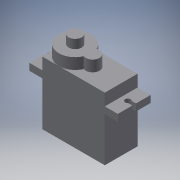
# Autodesk Inventor part: sg90
Saved by Autodesk Inventor 2018 (Build 220112000, 112)
## iProperties
Created: 2017-12-22
Part Number: sg90
Material: Generic
Document SubType Name: Modeling
Designer: Nirant Ramakuru
Density: 1 g/cm^3
Appearance: Default
Author: Nirant Ramakuru
Autodesk Inventor part; units mm, degrees
ref_plane "YZ Plane" through (0, 0, 0) normal (1, 0, 0) x (0, 1, 0)
ref_plane "XZ Plane" through (0, 0, 0) normal (0, 1, 0) x (-1, 0, 0)
ref_plane "XY Plane" through (0, 0, 0) normal (0, 0, 1) x (1, 0, 0)
sketch "Sketch1" plane through (0, 0, 0) normal (0, 1, 0) x (-1, 0, 0)
  line L0 (0, 0) -> (22.5, 0)
  line L1 (22.5, 0) -> (22.5, -11.8)
  line L2 (22.5, -11.8) -> (0, -11.8)
  line L3 (0, -11.8) -> (0, 0)
  dimension "d0" = 22.5
  dimension "d1" = 11.8
  constraints: 8 end point, 2 parallel, 1 horizontal, 1 perpendicular
  measures "d0" distance of L1.end L2.end
  measures "d1" distance of L0.end L1.end
extrude "Extrusion1" add sketch "Sketch1" along normal blind 22.7
sketch "Sketch2" plane through (0, 22.7, 0) normal (0, 1, 0) x (1, 0, 0)
  point P0 (0, 0)
sketch "Sketch3" plane through (0, 22.7, 0) normal (0, 1, 0) x (1, 0, 0)
  line L0 (-22.5, 0) -> (0, 0) projected
  line L1 (-18.5174, 0) -> (-18.5174, 5.9)
  line L2 (-18.5174, 0) -> (-12.6174, 0) construction
  line L3 (-22.5, 11.8) -> (-22.5, 0) projected
  line L4 (-22.5, 5.9) -> (-16.6, 5.9)
  circle A0 centre (-16.6, 5.9) radius 5.9
  dimension "d4" = 5.9
  dimension "d5" = 90
  dimension "d6" = 5.9
  constraints: 6 end point, 3 perpendicular, 1 coincident, 1 horizontal, 1 horizontal alignment, 1 midpoint, 1 point on line, 2 other
  measures "d4" distance of L1.start L1.end
  measures "d5" angle of L2 L1
  measures "d6" distance of L4.start L4.end
extrude "Extrusion2" add sketch "Sketch3" along normal blind 4 contours A0 L1 L4 | L4 L1 A0
sketch "Sketch4" plane through (0, 0, 0) normal (1, 0, 0) x (0, 0, -1)
  line L0 (0, 0) -> (11.8, 0) projected
  line L1 (5.9, 0) -> (5.9, 15.9)
  line L2 (0, 0) -> (0, 22.7) projected
  line L3 (11.8, 0) -> (11.8, 22.7) projected
  line L4 (0, 15.9) -> (11.8, 15.9)
  line L5 (11.8, 15.9) -> (11.8, 18.4)
  line L6 (11.8, 18.4) -> (0, 18.4)
  line L7 (0, 18.4) -> (0, 15.9)
  dimension "d9" = 15.9
  dimension "d10" = 2.5
  constraints: 10 end point, 2 parallel, 2 point on line, 1 horizontal, 1 midpoint, 1 perpendicular, 1 vertical
  measures "d9" distance of L1.start L1.end
  measures "d10" distance of L5.end L4.end
sketch "Sketch5" plane through (-22.5, 0, -11.8) normal (-1, 0, 0) x (0, 0, 1)
  line L0 (11.8, 0) -> (0, 0) projected
  line L1 (5.9, 0) -> (5.9, 15.9)
  line L2 (0, 0) -> (0, 22.7) projected
  line L3 (11.8, 0) -> (11.8, 22.7) projected
  line L4 (0, 15.9) -> (11.8, 15.9)
  line L5 (11.8, 15.9) -> (11.8, 18.4)
  line L6 (11.8, 18.4) -> (0, 18.4)
  line L7 (0, 18.4) -> (0, 15.9)
  dimension "d11" = 15.9
  dimension "d12" = 2.5
  constraints: 10 end point, 2 parallel, 2 point on line, 1 horizontal, 1 midpoint, 1 perpendicular, 1 vertical
  measures "d11" distance of L1.start L1.end
  measures "d12" distance of L5.end L4.end
extrude "Extrusion3" add sketch "Sketch5" along normal blind 4.7 contours L4 L2 L6 L3
extrude "Extrusion4" add sketch "Sketch4" along normal blind 4.7 contours L2 L6 L3 L4
sketch "Sketch6" plane through (-16.6, 26.7, -5.9) normal (0, 1, 0) x (1, 0, 0)
  point P0 (16.6, -5.9)
sketch "Sketch7" plane through (-16.6, 26.7, -5.9) normal (0, 1, 0) x (1, 0, 0)
  circle A0 centre (0, 0) radius 2.35
  point P0 (16.6, -5.9)
  dimension "d17" = 4.7
  constraints: 1 centre point, 1 coincident
  measures "d17" diameter of A0
extrude "Extrusion5" add sketch "Sketch7" along normal blind 3.2
sketch "Sketch8" plane through (0, 22.7, 0) normal (0, 1, 0) x (1, 0, 0)
  point P0 (0, 0)
sketch "Sketch9" plane through (-16.6, 26.7, -5.9) normal (0, 1, 0) x (1, 0, 0)
  line L0 (0, 0) -> (6.3, 0)
  point P0 (16.6, -5.9)
  dimension "d20" = 6.3
  constraints: 2 end point, 1 horizontal
  measures "d20" distance of L0.start L0.end
sketch "Sketch10" plane through (-16.6, 26.7, -5.9) normal (0, 1, 0) x (1, 0, 0)
  circle A0 centre (6.3, 0) radius 2.5
  point P0 (16.6, -5.9)
  dimension "d21" = 5
  constraints: 1 centre point
  measures "d21" diameter of A0
extrude "Extrusion6" add sketch "Sketch10" against normal blind 4
sketch "Sketch11" plane through (0, 18.4, 0) normal (0, 1, 0) x (1, 0, 0)
  line L0 (4.7, 0) -> (4.7, 11.8) projected
  line L1 (4.7, 5.9) -> (2.4, 5.9)
  circle A0 centre (2.4, 5.9) radius 1
  line L2 (0.1, 5.25) -> (4.7, 5.25)
  line L3 (4.7, 5.25) -> (4.7, 6.55)
  line L4 (4.7, 6.55) -> (0.1, 6.55)
  line L5 (0.1, 6.55) -> (0.1, 5.25)
  line L6 (2.4, 5.25) -> (2.4, 6.55)
  point P0 (0, 0)
  dimension "d24" = 2.3
  dimension "d25" = 2
  dimension "d26" = 1.3
  constraints: 12 end point, 3 midpoint, 2 horizontal, 2 parallel, 1 centre point, 1 coincident, 1 perpendicular, 1 point on line
  measures "d24" distance of L1.start L1.end
  measures "d25" diameter of A0
  measures "d26" distance of L3.end L2.end
extrude "Extrusion7" cut sketch "Sketch11" against normal blind 4 contours L2 L6 L1 A0 | A0 L2 | L1 L6 L4 A0 | A0 L4 L6 L2 | L4 A0
extrude "Extrusion8" cut sketch "Sketch11" against normal blind 4 contours L2 A0 L1 L0 | L1 A0 L4 L0 | L2 L6 L1 A0 | L1 L6 L4 A0
sketch "Sketch12" plane through (-22.5, 18.4, 0) normal (0, 1, 0) x (1, 0, 0)
  line L0 (-4.7, 0) -> (-4.7, 11.8) projected
  line L1 (-4.7, 5.9) -> (-2.4, 5.9)
  circle A0 centre (-2.4, 5.9) radius 1
  line L2 (-0.1, 5.25) -> (-4.7, 5.25)
  line L3 (-4.7, 5.25) -> (-4.7, 6.55)
  line L4 (-4.7, 6.55) -> (-0.1, 6.55)
  line L5 (-0.1, 6.55) -> (-0.1, 5.25)
  line L6 (-0.1, 5.25) -> (-4.7, 6.55) construction
  line L7 (-4.7, 5.25) -> (-0.1, 6.55) construction
  line L8 (-2.4, 5.25) -> (-2.4, 6.55)
  point P0 (22.5, 0)
  dimension "d31" = 2.3
  dimension "d32" = 2
  dimension "d33" = 1.3
  constraints: 16 end point, 5 midpoint, 2 horizontal, 2 parallel, 1 centre point, 1 coincident, 1 perpendicular, 1 point on line
  measures "d31" distance of L1.start L1.end
  measures "d32" diameter of A0
  measures "d33" distance of L2.end L3.end
extrude "Extrusion9" cut sketch "Sketch12" against normal blind 4 contours L0 L1 A0 L2 | L0 L4 A0 L1 | L2 A0 | A0 L1 L8 L2 | A0 L4 L8 L1 | L2 L8 L4 A0 | A0 L4
sketch "Sketch13" plane through (0, 0, 0) normal (0, -1, 0) x (1, 0, 0)
  point P0 (0, 0)
sketch "Sketch14" plane through (0, 18.4, 0) normal (0, 1, 0) x (1, 0, 0)
  arc A0 (3.1599, 6.55) -> (3.1599, 5.25) centre (2.4, 5.9) ccw projected
  line L0 (0, 0) -> (0, 11.8) projected
  dimension "d36" = 2.4
  dimension "d37" = 1
  measures "d36" distance from line of A0.centre L0
  measures "d37" radius of A0
body "Solid1"
